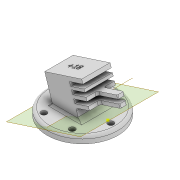
# Autodesk Inventor part: Plate_18
Saved by Autodesk Inventor 2022 (Build 260153000, 153)
## iProperties
Created: 2022-12-25
Part Number: Plate_18
Material: Generic
Document SubType Name: Modeling
Designer: dell
Density: 1 g/cm^3
Appearance: Default
Author: dell
Autodesk Inventor part; units mm, degrees
ref_plane "YZ Plane" through (0, 0, 0) normal (1, 0, 0) x (0, 1, 0)
ref_plane "XZ Plane" through (0, 0, 0) normal (0, 1, 0) x (-1, 0, 0)
ref_plane "XY Plane" through (0, 0, 0) normal (0, 0, 1) x (1, 0, 0)
sketch "Sketch1" plane through (0, 0, 0) normal (0, 1, 0) x (-1, 0, 0)
  circle A0 centre (0, 0) radius 50
  dimension "d0" = 100
  constraints: 1 centre point, 1 coincident
  measures "d0" diameter of A0
extrude "Extrusion1" add sketch "Sketch1" along normal blind 10
sketch "Sketch2" plane through (0, 10, 0) normal (0, 1, 0) x (1, 0, 0)
  circle A0 centre (-40, 0) radius 4.1
  point P0 (0, 0)
  dimension "d3" = 8.2
  dimension "d4" = 40
  constraints: 1 centre point
  measures "d3" diameter of A0
  measures "d4" distance of point (0, 0) A0.centre
extrude "Extrusion2" cut sketch "Sketch2" against normal blind 100
pattern_circular "Circular Pattern1" count 6 over 360 about axis through (0, 0, 0) along (0, 1, 0) of "Extrusion2"
ref_plane "Work Plane1" through (0, 10, -10) normal (0.309017, -0.9510565, 0) x (0, 0, 1)
sketch "Sketch3" plane through (0, 10, 0) normal (-0.309017, 0.9510565, 0) x (0.9510565, 0.309017, 0)
  line L0 (-20.5902, 20) -> (14.4098, 20)
  line L1 (14.4098, 20) -> (14.4098, -20)
  line L2 (14.4098, -20) -> (-20.5902, -20)
  line L3 (-20.5902, -20) -> (-20.5902, 20)
  line L4 (-20.5902, 20) -> (14.4098, -20) construction
  line L5 (14.4098, 20) -> (-20.5902, -20) construction
  point P0 (-3.0902, 0)
  dimension "d10" = 35
  dimension "d11" = 40
  constraints: 12 end point, 2 midpoint, 2 parallel, 1 horizontal, 1 perpendicular
  measures "d10" distance of L1.end L2.end
  measures "d11" distance of L0.end L1.end
extrude "Extrusion3" add sketch "Sketch3" along normal blind 45
sketch "Sketch5" plane through (15.1514, 10, 20) normal (0.9510565, 0.309017, 0) x (0, 0, -1)
  line L0 (0, 4.682) -> (0, 49.682) projected
  line L1 (40, 11.3722) -> (40, 49.682) projected
  line L2 (0, 19.682) -> (40, 19.682)
  line L3 (40, 19.682) -> (40, 14.682)
  line L4 (40, 14.682) -> (0, 14.682)
  line L5 (0, 14.682) -> (0, 19.682)
  line L6 (0, 11.3722) -> (0, 49.682) projected
  line L7 (0, 24.682) -> (40, 24.682)
  line L8 (40, 24.682) -> (40, 29.682)
  line L9 (40, 29.682) -> (0, 29.682)
  line L10 (0, 29.682) -> (0, 24.682)
  line L11 (40, 11.3722) -> (40, 49.682) projected
  line L12 (0, 38.882) -> (40, 38.882)
  line L13 (40, 38.882) -> (40, 34.682)
  line L14 (40, 34.682) -> (0, 34.682)
  line L15 (0, 34.682) -> (0, 38.882)
  line L16 (0, 43.882) -> (40, 43.882)
  line L17 (40, 4.682) -> (40, 49.682) projected
  line L18 (0, 49.682) -> (40, 49.682) projected
  line L19 (0, 4.682) -> (0, 49.682) projected
  line L20 (0, 4.682) -> (40, 4.682) projected
  point P0 (20, -4.8285)
  point P1 (0, 0)
  point P2 (0, 14.682)
  point P3 (40, 19.682)
  point P4 (0, 43.882)
  point P5 (40, 43.882)
  point P6 (0, 34.682)
  point P7 (40, 34.682)
  point P8 (40, 38.882)
  point P9 (0, 38.882)
  point P10 (0, 29.682)
  point P11 (0, 24.682)
  point P12 (40, 24.682)
  dimension "d16" = 5
  dimension "d19" = 5
  dimension "d20" = 5
  dimension "d21" = 5
  dimension "d22" = 4.2
  dimension "d23" = 5
  dimension "d44" = 15
  constraints: 26 end point, 8 point on line, 6 parallel, 4 perpendicular, 3 horizontal
  measures "d16" distance between parallel lines of L2 L4
  measures "d19" distance between parallel lines of L7 L2
  measures "d20" distance between parallel lines of L7 L9
  measures "d21" distance between parallel lines of L9 L14
  measures "d22" distance between parallel lines of L14 L12
  measures "d23" distance between parallel lines of L12 L16
  measures "d44" distance between parallel lines of L20 L2
extrude "Extrusion4" add sketch "Sketch5" along normal blind 20 contours L0 L2 L1 L4 | L0 L9 L1 L7 | L0 L12 L1 L14 | L0 L18 L1 L16
sketch "Sketch7" plane through (34.1725, 16.1803, 20) normal (0.9510565, 0.309017, 0) x (0, 0, -1)
  point P0 (20, -4.8285)
sketch "Sketch6" plane through (34.1725, 16.1803, 20) normal (0.9510565, 0.309017, 0) x (0, 0, -1)
  line L0 (40, 14.682) -> (40, 19.682) projected
  line L1 (40, 19.682) -> (0, 19.682) projected
  line L2 (0, 19.682) -> (0, 14.682) projected
  line L3 (0, 14.682) -> (40, 14.682) projected
  line L4 (0, 29.682) -> (0, 24.682) projected
  line L5 (0, 24.682) -> (40, 24.682) projected
  line L6 (40, 24.682) -> (40, 29.682) projected
  line L7 (40, 29.682) -> (0, 29.682) projected
  line L8 (40, 29.682) -> (0, 29.682) projected
  line L9 (15.5, 29.682) -> (24.5, 29.682)
  line L10 (24.5, 29.682) -> (24.5, 24.682)
  line L11 (24.5, 24.682) -> (15.5, 24.682)
  line L12 (15.5, 24.682) -> (15.5, 29.682)
  line L13 (40, 19.682) -> (0, 19.682) projected
  line L14 (15.5, 19.682) -> (24.5, 19.682)
  line L15 (24.5, 19.682) -> (24.5, 14.682)
  line L16 (24.5, 14.682) -> (15.5, 14.682)
  line L17 (15.5, 14.682) -> (15.5, 19.682)
  line L18 (20, -38.525) -> (20, 89.1942) projected
  point P0 (20, -4.8285)
  point P1 (15.5, 14.682)
  point P2 (24.5, 29.682)
  point P3 (15.5, 29.682)
  dimension "d24" = 9
  dimension "d25" = 9
  dimension "d26" = 4.5
  dimension "d27" = 4.5
  constraints: 16 end point, 4 parallel, 4 point on line, 2 horizontal, 2 perpendicular
  measures "d24" distance between parallel lines of L10 L12
  measures "d25" distance between parallel lines of L17 L15
  measures "d26" distance between parallel lines of L18 L12
  measures "d27" distance between parallel lines of L18 L17
extrude "Extrusion5" add sketch "Sketch6" along normal blind 30 contours L3 L18 L1 L15 | L3 L17 L1 L18 | L7 L18 L5 L12 | L7 L10 L5 L18
thicken "Thicken1" operation add thickness 0.2 both sides no extend neighbours yes toward (0.309017, -0.9510565, 0) faces at (15.4097, 30.7788, -1.5)
thicken "Thicken2" operation add thickness 0.2 both sides no extend neighbours yes toward (-0.309017, 0.9510565, 0) faces at (13.8646, 35.5341, -1.5)
thicken "Thicken3" operation add thickness 0.2 both sides no extend neighbours yes toward (0.309017, -0.9510565, 0) faces at (12.3195, 40.2894, 1.5)
thicken "Thicken4" operation add thickness 0.2 both sides no extend neighbours yes toward (-0.309017, 0.9510565, 0) faces at (10.7744, 45.0447, 6.6667)
thicken "Thicken5" operation add thickness 0.2 both sides no extend neighbours yes toward (0.309017, -0.9510565, 0) faces at (15.8169, 51.0992, 6.6667)
thicken "Thicken6" operation add thickness 0.2 both sides no extend neighbours yes toward (-0.309017, 0.9510565, 0) faces at (7.9315, 53.7944, -6.6667)
fillet "Fillet1" radius 3 8 edges at (-21.6498, 10, 0) (-10.8249, 10, -20) (-10.8249, 10, 20) (10.6144, 23.9634, 0) (28.8939, 32.4263, -4.5) (25.7728, 42.032, -4.5) (25.7728, 42.032, 4.5) (28.8939, 32.4263, 4.5)
chamfer "Chamfer1" distance 14 angle 45 3 edges at (0, 10, -21.5) (0, 10, 0) (0, 10, 21.5)
fillet "Fillet3" radius 10 3 edges at (14, 10, 0) (14, 10, 21.5) (14, 10, -21.5)
fillet "Fillet4" radius 4 1 edges at (50, 10, 0)
sketch "Sketch8" plane through (-13.9058, 52.7975, 0) normal (-0.309017, 0.9510565, 0) x (0.9510565, 0.309017, 0)
  line L0 (-6.9685, 4.6888) -> (10.8183, 4.6888) construction
  line L1 (10.8183, 4.6888) -> (10.8183, -13.2224) construction
  line L2 (10.8183, -13.2224) -> (-6.9685, -13.2224) construction
  line L3 (-6.9685, -13.2224) -> (-6.9685, 4.6888) construction
  line L4 (0.1952, -0.4198) -> (-2.5147, -0.4198)
  line L5 (-2.5147, -0.4198) -> (-2.5147, -3.1297)
  line L6 (-2.5147, -3.1297) -> (-3.4093, -3.1297)
  line L7 (-3.4093, -3.1297) -> (-3.4093, -0.4198)
  line L8 (-3.4093, -0.4198) -> (-6.1192, -0.4198)
  line L9 (-6.1192, -0.4198) -> (-6.1192, 0.4424)
  line L10 (-6.1192, 0.4424) -> (-3.4093, 0.4424)
  line L11 (-3.4093, 0.4424) -> (-3.4093, 3.1523)
  line L12 (-3.4093, 3.1523) -> (-2.5147, 3.1523)
  line L13 (-2.5147, 3.1523) -> (-2.5147, 0.4424)
  line L14 (-2.5147, 0.4424) -> (0.1952, 0.4424)
  line L15 (0.1952, 0.4424) -> (0.1952, -0.4198)
  line L16 (6.1531, -3.4928) -> (2.2503, -3.4928)
  line L17 (2.2503, -3.4928) -> (2.2503, -2.6759)
  line L18 (2.2503, -2.6759) -> (3.7025, -2.6759)
  line L19 (3.7025, -2.6759) -> (3.7025, 2.6855)
  line L20 (3.7025, 2.6855) -> (2.2503, 2.6855)
  line L21 (2.2503, 2.6855) -> (2.2503, 3.4181)
  spline S0 degree 2 poles (2.2503, 3.4181) (3.0736, 3.4181) (3.8516, 3.8849) (3.9035, 4.5332) knots 0 0 0 1 2 2 2
  line L22 (3.9035, 4.5332) -> (4.7333, 4.5332)
  line L23 (4.7333, 4.5332) -> (4.7333, -2.6759)
  line L24 (4.7333, -2.6759) -> (6.1531, -2.6759)
  line L25 (6.1531, -2.6759) -> (6.1531, -3.4928)
  spline S1 degree 2 poles (10.0428, -3.6743) (9.4464, -3.6743) (8.4675, -3.3177) (8.1239, -2.9871) knots 0 0 0 1 2 2 2
  spline S2 degree 2 poles (8.1239, -2.9871) (7.7868, -2.6629) (7.4367, -1.7813) (7.4367, -1.2821) knots 0 0 0 1 2 2 2
  spline S3 degree 2 poles (7.4367, -1.2821) (7.4367, -0.6338) (8.1304, 0.4554) (8.7916, 0.7795) knots 0 0 0 1 2 2 2
  line L26 (8.7916, 0.7795) -> (8.7916, 0.8119)
  spline S4 degree 2 poles (8.7916, 0.8119) (8.2017, 1.1555) (7.6312, 1.9724) (7.6312, 2.5818) knots 0 0 0 1 2 2 2
  spline S5 degree 2 poles (7.6312, 2.5818) (7.6312, 3.4829) (8.9926, 4.6888) (10.0428, 4.6888) knots 0 0 0 1 2 2 2
  spline S6 degree 2 poles (10.0428, 4.6888) (11.132, 4.6888) (12.448, 3.5478) (12.448, 2.6531) knots 0 0 0 1 2 2 2
  spline S7 degree 2 poles (12.448, 2.6531) (12.448, 2.115) (11.8192, 1.0648) (11.2292, 0.7666) knots 0 0 0 1 2 2 2
  line L27 (11.2292, 0.7666) -> (11.2292, 0.7341)
  spline S8 degree 2 poles (11.2292, 0.7341) (11.9294, 0.41) (12.649, -0.5236) (12.649, -1.2626) knots 0 0 0 1 2 2 2
  spline S9 degree 2 poles (12.649, -1.2626) (12.649, -2.2869) (11.1579, -3.6743) (10.0428, -3.6743) knots 0 0 0 1 2 2 2
  spline S10 degree 2 poles (11.5469, -1.3663) (11.5469, -0.8736) (11.1579, -0.2902) (10.6069, 0.0081) knots 0 0 0 1 2 2 2
  spline S11 degree 2 poles (10.6069, 0.0081) (10.4253, 0.1118) (9.8159, 0.3516) (9.4334, 0.5072) knots 0 0 0 1 2 2 2
  spline S12 degree 2 poles (9.4334, 0.5072) (8.9926, 0.2155) (8.5193, -0.6532) (8.5193, -1.2043) knots 0 0 0 1 2 2 2
  spline S13 degree 2 poles (8.5193, -1.2043) (8.5193, -1.9304) (9.3945, -2.8769) (10.0558, -2.8769) knots 0 0 0 1 2 2 2
  spline S14 degree 2 poles (10.0558, -2.8769) (10.73, -2.8769) (11.5469, -2.0665) (11.5469, -1.3663) knots 0 0 0 1 2 2 2
  spline S15 degree 2 poles (11.3978, 2.6401) (11.3978, 3.1782) (10.6782, 3.8978) (10.0364, 3.8978) knots 0 0 0 1 2 2 2
  spline S16 degree 2 poles (10.0364, 3.8978) (9.4529, 3.8978) (8.7074, 3.256) (8.7074, 2.705) knots 0 0 0 1 2 2 2
  spline S17 degree 2 poles (8.7074, 2.705) (8.7074, 2.3095) (9.0898, 1.7585) (9.4723, 1.538) knots 0 0 0 1 2 2 2
  spline S18 degree 2 poles (9.4723, 1.538) (9.6344, 1.4473) (10.3216, 1.1296) (10.6004, 1.0388) knots 0 0 0 1 2 2 2
  spline S19 degree 2 poles (10.6004, 1.0388) (11.0672, 1.3954) (11.3978, 2.1539) (11.3978, 2.6401) knots 0 0 0 1 2 2 2
  point P0 (-3.0902, 0)
  constraints: 2 other
extrude "Extrusion6" cut sketch "Sketch8" against normal blind 1
fillet "Fillet5" radius 1 4 edges at (57.4256, 41.6968, 4.5) (54.3045, 51.3025, 4.5) (54.3045, 51.3025, -4.5) (57.4256, 41.6968, -4.5)
equation "\"d26\" = 0.5 * d24"
equation "\"d27\" = 0.5 * d25"
body "Solid1"
